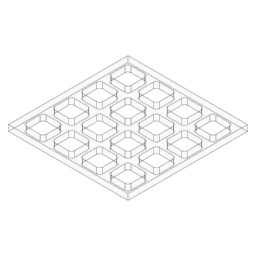
SynthBox v1 (Autodesk Fusion 360 design; units mm, degrees)
Autodesk Fusion 360 part; units mm, degrees
sketch "Sketch1" plane through (0, 0, 0) normal (0, 0, 1) x (1, 0, 0)
  line L0 (0, 0) -> (60, 0)
  line L1 (60, 0) -> (60, 60)
  line L2 (60, 60) -> (0, 60)
  line L3 (0, 60) -> (0, 0)
  arc A0 (0, 124.28) -> (0, 185.3988) centre (-137.08, 154.8394) ccw
  line L4 (30, 60) -> (30, 0) construction
  line L5 (0, 30) -> (60, 30) construction
  line L6 (30, 30) -> (32.1, 30) construction
  line L7 (32.1, 30) -> (32.1, 32.1) construction
  line L8 (32.1, 40.6) -> (32.1, 33.6)
  line L9 (33.6, 32.1) -> (40.6, 32.1)
  line L10 (42.1, 33.6) -> (42.1, 40.6)
  line L11 (42.1, 42.1) -> (40.6, 42.1) construction
  line L12 (40.6, 42.1) -> (33.6, 42.1)
  arc A1 (40.6, 32.1) -> (42.1, 33.6) centre (40.6, 33.6) ccw
  arc A2 (42.1, 40.6) -> (40.6, 42.1) centre (40.6, 40.6) ccw
  line L13 (32.1, 42.1) -> (32.1, 40.6) construction
  arc A3 (33.6, 42.1) -> (32.1, 40.6) centre (33.6, 40.6) ccw
  arc A4 (32.1, 33.6) -> (33.6, 32.1) centre (33.6, 33.6) ccw
  line L14 (42.1, 33.6) -> (42.1, 40.6)
  arc A5 (42.1, 40.6) -> (40.6, 42.1) centre (40.6, 40.6) ccw
  line L15 (40.6, 42.1) -> (33.6, 42.1)
  arc A6 (33.6, 42.1) -> (32.1, 40.6) centre (33.6, 40.6) ccw
  line L16 (32.1, 40.6) -> (32.1, 33.6)
  arc A7 (32.1, 33.6) -> (33.6, 32.1) centre (33.6, 33.6) ccw
  line L17 (17.9, 40.6) -> (17.9, 33.6)
  arc A8 (19.4, 42.1) -> (17.9, 40.6) centre (19.4, 40.6) ccw
  line L18 (26.4, 42.1) -> (19.4, 42.1)
  arc A9 (27.9, 40.6) -> (26.4, 42.1) centre (26.4, 40.6) ccw
  line L19 (27.9, 33.6) -> (27.9, 40.6)
  arc A10 (26.4, 32.1) -> (27.9, 33.6) centre (26.4, 33.6) ccw
  line L20 (19.4, 32.1) -> (26.4, 32.1)
  arc A11 (17.9, 33.6) -> (19.4, 32.1) centre (19.4, 33.6) ccw
  line L21 (12.2, 42.1) -> (5.2, 42.1)
  line L22 (3.7, 40.6) -> (3.7, 33.6)
  arc A12 (13.7, 40.6) -> (12.2, 42.1) centre (12.2, 40.6) ccw
  arc A13 (12.2, 32.1) -> (13.7, 33.6) centre (12.2, 33.6) ccw
  arc A14 (5.2, 42.1) -> (3.7, 40.6) centre (5.2, 40.6) ccw
  line L23 (5.2, 32.1) -> (12.2, 32.1)
  arc A15 (3.7, 33.6) -> (5.2, 32.1) centre (5.2, 33.6) ccw
  line L24 (13.7, 33.6) -> (13.7, 40.6)
  arc A16 (56.3, 40.6) -> (54.8, 42.1) centre (54.8, 40.6) ccw
  line L25 (47.8, 32.1) -> (54.8, 32.1)
  arc A17 (54.8, 32.1) -> (56.3, 33.6) centre (54.8, 33.6) ccw
  line L26 (54.8, 42.1) -> (47.8, 42.1)
  line L27 (56.3, 33.6) -> (56.3, 40.6)
  arc A18 (46.3, 33.6) -> (47.8, 32.1) centre (47.8, 33.6) ccw
  line L28 (46.3, 40.6) -> (46.3, 33.6)
  arc A19 (47.8, 42.1) -> (46.3, 40.6) centre (47.8, 40.6) ccw
  line L29 (27.9, 47.8) -> (27.9, 54.8)
  line L30 (17.9, 54.8) -> (17.9, 47.8)
  arc A20 (12.2, 46.3) -> (13.7, 47.8) centre (12.2, 47.8) ccw
  line L31 (3.7, 54.8) -> (3.7, 47.8)
  arc A21 (3.7, 47.8) -> (5.2, 46.3) centre (5.2, 47.8) ccw
  line L32 (12.2, 56.3) -> (5.2, 56.3)
  arc A22 (27.9, 54.8) -> (26.4, 56.3) centre (26.4, 54.8) ccw
  line L33 (26.4, 56.3) -> (19.4, 56.3)
  arc A23 (5.2, 56.3) -> (3.7, 54.8) centre (5.2, 54.8) ccw
  line L34 (19.4, 46.3) -> (26.4, 46.3)
  line L35 (5.2, 46.3) -> (12.2, 46.3)
  arc A24 (19.4, 56.3) -> (17.9, 54.8) centre (19.4, 54.8) ccw
  arc A25 (13.7, 54.8) -> (12.2, 56.3) centre (12.2, 54.8) ccw
  arc A26 (26.4, 46.3) -> (27.9, 47.8) centre (26.4, 47.8) ccw
  arc A27 (17.9, 47.8) -> (19.4, 46.3) centre (19.4, 47.8) ccw
  line L36 (13.7, 47.8) -> (13.7, 54.8)
  arc A28 (32.1, 47.8) -> (33.6, 46.3) centre (33.6, 47.8) ccw
  arc A29 (40.6, 46.3) -> (42.1, 47.8) centre (40.6, 47.8) ccw
  arc A30 (33.6, 56.3) -> (32.1, 54.8) centre (33.6, 54.8) ccw
  arc A31 (54.8, 46.3) -> (56.3, 47.8) centre (54.8, 47.8) ccw
  line L37 (46.3, 54.8) -> (46.3, 47.8)
  line L38 (56.3, 47.8) -> (56.3, 54.8)
  line L39 (42.1, 47.8) -> (42.1, 54.8)
  line L40 (32.1, 54.8) -> (32.1, 47.8)
  line L41 (33.6, 46.3) -> (40.6, 46.3)
  arc A32 (46.3, 47.8) -> (47.8, 46.3) centre (47.8, 47.8) ccw
  line L42 (47.8, 46.3) -> (54.8, 46.3)
  arc A33 (47.8, 56.3) -> (46.3, 54.8) centre (47.8, 54.8) ccw
  line L43 (54.8, 56.3) -> (47.8, 56.3)
  line L44 (40.6, 56.3) -> (33.6, 56.3)
  arc A34 (42.1, 54.8) -> (40.6, 56.3) centre (40.6, 54.8) ccw
  arc A35 (56.3, 54.8) -> (54.8, 56.3) centre (54.8, 54.8) ccw
  arc A36 (56.3, 26.4) -> (54.8, 27.9) centre (54.8, 26.4) ccw
  line L45 (26.4, 27.9) -> (19.4, 27.9)
  arc A37 (27.9, 26.4) -> (26.4, 27.9) centre (26.4, 26.4) ccw
  line L46 (54.8, 27.9) -> (47.8, 27.9)
  line L47 (3.7, 26.4) -> (3.7, 19.4)
  arc A38 (26.4, 17.9) -> (27.9, 19.4) centre (26.4, 19.4) ccw
  line L48 (47.8, 17.9) -> (54.8, 17.9)
  arc A39 (17.9, 19.4) -> (19.4, 17.9) centre (19.4, 19.4) ccw
  arc A40 (40.6, 17.9) -> (42.1, 19.4) centre (40.6, 19.4) ccw
  line L49 (12.2, 27.9) -> (5.2, 27.9)
  arc A41 (13.7, 26.4) -> (12.2, 27.9) centre (12.2, 26.4) ccw
  line L50 (13.7, 19.4) -> (13.7, 26.4)
  arc A42 (5.2, 27.9) -> (3.7, 26.4) centre (5.2, 26.4) ccw
  line L51 (33.6, 17.9) -> (40.6, 17.9)
  line L52 (42.1, 19.4) -> (42.1, 26.4)
  arc A43 (42.1, 26.4) -> (40.6, 27.9) centre (40.6, 26.4) ccw
  line L53 (27.9, 19.4) -> (27.9, 26.4)
  arc A44 (54.8, 17.9) -> (56.3, 19.4) centre (54.8, 19.4) ccw
  line L54 (56.3, 19.4) -> (56.3, 26.4)
  arc A45 (33.6, 27.9) -> (32.1, 26.4) centre (33.6, 26.4) ccw
  arc A46 (47.8, 27.9) -> (46.3, 26.4) centre (47.8, 26.4) ccw
  line L55 (46.3, 26.4) -> (46.3, 19.4)
  arc A47 (46.3, 19.4) -> (47.8, 17.9) centre (47.8, 19.4) ccw
  arc A48 (3.7, 19.4) -> (5.2, 17.9) centre (5.2, 19.4) ccw
  line L56 (40.6, 27.9) -> (33.6, 27.9)
  arc A49 (12.2, 17.9) -> (13.7, 19.4) centre (12.2, 19.4) ccw
  arc A50 (19.4, 27.9) -> (17.9, 26.4) centre (19.4, 26.4) ccw
  line L57 (32.1, 26.4) -> (32.1, 19.4)
  line L58 (5.2, 17.9) -> (12.2, 17.9)
  line L59 (17.9, 26.4) -> (17.9, 19.4)
  arc A51 (32.1, 19.4) -> (33.6, 17.9) centre (33.6, 19.4) ccw
  line L60 (19.4, 17.9) -> (26.4, 17.9)
  line L61 (26.4, 13.7) -> (19.4, 13.7)
  line L62 (3.7, 12.2) -> (3.7, 5.2)
  line L63 (13.7, 5.2) -> (13.7, 12.2)
  arc A52 (47.8, 13.7) -> (46.3, 12.2) centre (47.8, 12.2) ccw
  arc A53 (40.6, 3.7) -> (42.1, 5.2) centre (40.6, 5.2) ccw
  arc A54 (13.7, 12.2) -> (12.2, 13.7) centre (12.2, 12.2) ccw
  arc A55 (33.6, 13.7) -> (32.1, 12.2) centre (33.6, 12.2) ccw
  arc A56 (32.1, 5.2) -> (33.6, 3.7) centre (33.6, 5.2) ccw
  line L64 (54.8, 13.7) -> (47.8, 13.7)
  line L65 (27.9, 5.2) -> (27.9, 12.2)
  line L66 (47.8, 3.7) -> (54.8, 3.7)
  arc A57 (3.7, 5.2) -> (5.2, 3.7) centre (5.2, 5.2) ccw
  arc A58 (42.1, 12.2) -> (40.6, 13.7) centre (40.6, 12.2) ccw
  line L67 (33.6, 3.7) -> (40.6, 3.7)
  arc A59 (27.9, 12.2) -> (26.4, 13.7) centre (26.4, 12.2) ccw
  line L68 (56.3, 5.2) -> (56.3, 12.2)
  arc A60 (54.8, 3.7) -> (56.3, 5.2) centre (54.8, 5.2) ccw
  line L69 (19.4, 3.7) -> (26.4, 3.7)
  line L70 (32.1, 12.2) -> (32.1, 5.2)
  arc A61 (56.3, 12.2) -> (54.8, 13.7) centre (54.8, 12.2) ccw
  line L71 (42.1, 5.2) -> (42.1, 12.2)
  arc A62 (46.3, 5.2) -> (47.8, 3.7) centre (47.8, 5.2) ccw
  line L72 (40.6, 13.7) -> (33.6, 13.7)
  line L73 (46.3, 12.2) -> (46.3, 5.2)
  arc A63 (19.4, 13.7) -> (17.9, 12.2) centre (19.4, 12.2) ccw
  arc A64 (26.4, 3.7) -> (27.9, 5.2) centre (26.4, 5.2) ccw
  line L74 (12.2, 13.7) -> (5.2, 13.7)
  arc A65 (12.2, 3.7) -> (13.7, 5.2) centre (12.2, 5.2) ccw
  line L75 (17.9, 12.2) -> (17.9, 5.2)
  line L76 (5.2, 3.7) -> (12.2, 3.7)
  arc A66 (5.2, 13.7) -> (3.7, 12.2) centre (5.2, 12.2) ccw
  arc A67 (17.9, 5.2) -> (19.4, 3.7) centre (19.4, 5.2) ccw
  point P0 (33.6, 32.1)
  point P1 (32.1, 33.6)
  point P2 (40.6, 32.1)
  point P3 (42.1, 33.6)
  point P4 (42.1, 40.6)
  dimension "d1" = 60
  dimension "d2" = 60
  dimension "d3" = 2.1
  dimension "d4" = 2.1
  dimension "d8" = 1.5
  dimension "d21" = 7
  dimension "d22" = 7
  dimension "d25" = 7
  dimension "d29" = 1.5
  dimension "d30" = 1.5
  dimension "d32" = 1.5
  dimension "d33" = 1.5
  dimension "d34" = 1.5
  dimension "d35" = 1.5
  dimension "d36" = 1.5
  dimension "d37" = 1.5
  dimension "d38" = 1.5
  dimension "d39" = 1.5
  dimension "d40" = 1.5
  dimension "d41" = 1.5
  dimension "d42" = 1.5
  dimension "d43" = 1.5
  dimension "d44" = 1.5
  dimension "d45" = 1.5
  dimension "d46" = 1.5
  dimension "d47" = 1.5
  dimension "d48" = 1.5
  dimension "d49" = 1.5
  dimension "d50" = 1.5
  dimension "d51" = 1.5
  dimension "d52" = 1.5
  dimension "d53" = 1.5
  dimension "d54" = 1.5
  dimension "d55" = 1.5
  dimension "d56" = 1.5
  dimension "d57" = 1.5
  dimension "d58" = 1.5
  dimension "d59" = 1.5
  dimension "d60" = 1.5
  dimension "d61" = 1.5
  dimension "d62" = 1.5
  dimension "d63" = 1.5
  dimension "d64" = 1.5
  dimension "d65" = 1.5
  dimension "d66" = 1.5
  dimension "d67" = 1.5
  dimension "d68" = 1.5
  dimension "d69" = 1.5
  dimension "d70" = 1.5
  dimension "d71" = 1.5
  dimension "d72" = 1.5
  dimension "d73" = 1.5
  dimension "d74" = 1.5
  dimension "d75" = 1.5
  dimension "d76" = 1.5
  dimension "d77" = 1.5
  dimension "d78" = 1.5
  dimension "d79" = 1.5
  dimension "d80" = 1.5
  dimension "d81" = 1.5
  dimension "d82" = 1.5
  dimension "d83" = 1.5
  dimension "d84" = 1.5
  dimension "d85" = 1.5
  dimension "d86" = 1.5
  dimension "d87" = 1.5
  dimension "d88" = 1.5
  dimension "d89" = 1.5
  dimension "d90" = 1.5
  dimension "d91" = 1.5
  dimension "d92" = 1.5
  dimension "d93" = 1.5
  dimension "d94" = 1.5
  dimension "d95" = 1.5
  dimension "d96" = 1.5
  constraint horizontal L0
  constraint vertical L1
  constraint horizontal L2
  constraint vertical L3
  constraint coincident L0.start L3.end
  constraint midpoint L2 L4.start
  constraint midpoint L0 L4.end
  constraint midpoint L3 L5.start
  constraint midpoint L1 L5.end
  constraint midpoint L5 L6.start
  constraint perpendicular L4 L6
  constraint perpendicular L5 L7
  constraint parallel L11 L12
  constraint coincident P2 L9
  constraint coincident P3 L10
  constraint tangent L9 A1
  constraint tangent L10 A1
  constraint coincident P4 L10
  constraint coincident L11.end L12
  constraint tangent L10 A2
  constraint tangent L12 A2
  constraint coincident L13.end L8
  constraint tangent L12 A3
  constraint tangent L8 A3
  constraint coincident P1 L8
  constraint coincident P0 L9
  constraint tangent L8 A4
  constraint tangent L9 A4
  constraint tangent L14 A5
  constraint tangent A5 L15
  constraint tangent L15 A6
  constraint tangent A6 L16
  constraint tangent L16 A7
  constraint tangent A10 L20
  constraint tangent L19 A10
  constraint tangent L17 A8
  constraint tangent L17 A11
  constraint tangent L20 A11
  constraint tangent L18 A9
  constraint tangent A13 L23
  constraint tangent A13 L24
  constraint tangent L22 A14
  constraint tangent L22 A15
  constraint tangent L23 A15
  constraint tangent L21 A12
  constraint tangent L25 A17
  constraint tangent A17 L27
  constraint tangent L28 A19
  constraint tangent A18 L28
  constraint tangent L25 A18
  constraint tangent A16 L26
  constraint tangent L34 A26
  constraint tangent L29 A26
  constraint tangent L30 A24
  constraint tangent L30 A27
  constraint tangent L34 A27
  constraint tangent A22 L33
  constraint tangent A20 L35
  constraint tangent A20 L36
  constraint tangent L31 A23
  constraint tangent L31 A21
  constraint tangent A21 L35
  constraint tangent L32 A25
  constraint tangent A31 L42
  constraint tangent A31 L38
  constraint tangent L37 A33
  constraint tangent L37 A32
  constraint tangent A32 L42
  constraint tangent L43 A35
  constraint tangent A29 L41
  constraint tangent A29 L39
  constraint tangent A30 L40
  constraint tangent A28 L40
  constraint tangent A28 L41
  constraint tangent L44 A34
  constraint tangent A38 L60
  constraint tangent A38 L53
  constraint tangent A50 L59
  constraint tangent A39 L59
  constraint tangent A39 L60
  constraint tangent L45 A37
  constraint tangent A49 L58
  constraint tangent L50 A49
  constraint tangent L47 A42
  constraint tangent L47 A48
  constraint tangent A48 L58
  constraint tangent L49 A41
  constraint tangent L48 A44
  constraint tangent A44 L54
  constraint tangent A46 L55
  constraint tangent L55 A47
  constraint tangent L48 A47
  constraint tangent A36 L46
  constraint tangent A40 L51
  constraint tangent A40 L52
  constraint tangent A45 L57
  constraint tangent L57 A51
  constraint tangent L51 A51
  constraint tangent A43 L56
  constraint tangent L69 A64
  constraint tangent L65 A64
  constraint tangent A63 L75
  constraint tangent L75 A67
  constraint tangent L69 A67
  constraint tangent L61 A59
  constraint tangent A65 L76
  constraint tangent L63 A65
  constraint tangent L62 A66
  constraint tangent L62 A57
  constraint tangent A57 L76
  constraint tangent A54 L74
  constraint tangent L66 A60
  constraint tangent L68 A60
  constraint tangent A52 L73
  constraint tangent A62 L73
  constraint tangent L66 A62
  constraint tangent L64 A61
  constraint tangent A53 L67
  constraint tangent A53 L71
  constraint tangent A55 L70
  constraint tangent A56 L70
  constraint tangent A56 L67
  constraint tangent A58 L72
  measures "d1" distance of L0.start L0.end
  measures "d2" distance of L0.start L2.end
  measures "d3" distance of L6.start L6.end
  measures "d4" distance of L6.end L7.end
  measures "d8" distance of L7.end P0
  measures "d21" distance of L8.start P1
  measures "d22" distance of P0 P2
  measures "d25" distance of P3 P4
  measures "d29" radius of A1
  measures "d30" radius of A2
  measures "d32" radius of A3
  measures "d33" radius of A4
  measures "d34" radius of A5
  measures "d35" radius of A6
  measures "d36" radius of A7
  measures "d37" radius of A10
  measures "d38" radius of A8
  measures "d39" radius of A11
  measures "d40" radius of A9
  measures "d41" radius of A13
  measures "d42" radius of A14
  measures "d43" radius of A15
  measures "d44" radius of A12
  measures "d45" radius of A17
  measures "d46" radius of A19
  measures "d47" radius of A18
  measures "d48" radius of A16
  measures "d49" radius of A26
  measures "d50" radius of A24
  measures "d51" radius of A27
  measures "d52" radius of A22
  measures "d53" radius of A20
  measures "d54" radius of A23
  measures "d55" radius of A21
  measures "d56" radius of A25
  measures "d57" radius of A31
  measures "d58" radius of A33
  measures "d59" radius of A32
  measures "d60" radius of A35
  measures "d61" radius of A29
  measures "d62" radius of A30
  measures "d63" radius of A28
  measures "d64" radius of A34
  measures "d65" radius of A38
  measures "d66" radius of A50
  measures "d67" radius of A39
  measures "d68" radius of A37
  measures "d69" radius of A49
  measures "d70" radius of A42
  measures "d71" radius of A48
  measures "d72" radius of A41
  measures "d73" radius of A44
  measures "d74" radius of A46
  measures "d75" radius of A47
  measures "d76" radius of A36
  measures "d77" radius of A40
  measures "d78" radius of A45
  measures "d79" radius of A51
  measures "d80" radius of A43
  measures "d81" radius of A64
  measures "d82" radius of A63
  measures "d83" radius of A67
  measures "d84" radius of A59
  measures "d85" radius of A65
  measures "d86" radius of A66
  measures "d87" radius of A57
  measures "d88" radius of A54
  measures "d89" radius of A60
  measures "d90" radius of A52
  measures "d91" radius of A62
  measures "d92" radius of A61
  measures "d93" radius of A53
  measures "d94" radius of A55
  measures "d95" radius of A56
  measures "d96" radius of A58
extrude "Extrude1" add sketch "Sketch1" along normal blind 5
extrude "Extrude2" cut 1 faces at (58.7667, 31.2, 5) along direction (0, 0, -1) blind 2
component "TopPlateGrid1" placed x (1, 0, 0) y (0, 1, 0) z (0, 0, 1) at (0, 0, 0)
